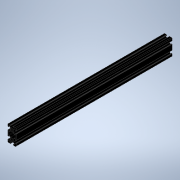
# Autodesk Inventor part: 2020 Aluminium Extrusion European Standard
Saved by Autodesk Inventor 2020 (Build 240168000, 168)
## iProperties
Created: 2019-10-16
Part Number: 2020 Aluminium Extrusion European Standard
Material: Generic
Document SubType Name: Modeling
Designer: Johnson Ebenezer R
Density: 1 g/cm^3
Appearance: Anodized - Black
Author: Johnson Ebenezer R
## iProperties of the stored document _3DPrint.ipt
Created: 2019-10-16
Part Number: _3DPrint
Material: Generic
Document SubType Name: Modeling
Designer: Johnson Ebenezer R
Density: 1 g/cm^3
Appearance: Default
Author: Johnson Ebenezer R
Autodesk Inventor part; units mm, degrees
ref_plane "YZ Plane" through (0, 0, 0) normal (1, 0, 0) x (0, 1, 0)
ref_plane "XZ Plane" through (0, 0, 0) normal (0, 1, 0) x (-1, 0, 0)
ref_plane "XY Plane" through (0, 0, 0) normal (0, 0, 1) x (1, 0, 0)
sketch "Sketch1" plane through (0, 0, 0) normal (0, 0, 1) x (1, 0, 0)
  line L0 (-10, -10) -> (10, -10) construction
  line L1 (10, -10) -> (10, 10) construction
  line L2 (10, 10) -> (-10, 10) construction
  line L3 (-10, 10) -> (-10, -10) construction
  line L4 (-10, -10) -> (10, 10) construction
  line L5 (10, -10) -> (-10, 10) construction
  line L6 (-10, 0) -> (10, 0) construction
  line L7 (-3.6, -10) -> (-10, -10)
  line L8 (-10, -10) -> (-10, -3.6)
  line L9 (3.6, -10) -> (10, -10)
  line L10 (10, -10) -> (10, -3.6)
  line L11 (-3.6, -10) -> (-3.6, -9.1)
  line L12 (3.6, -10) -> (3.6, -9.1)
  line L13 (-3.6, -9.1) -> (-3.1, -9.1)
  line L14 (-3.1, -9.1) -> (-3.1, -8.2)
  line L15 (3.6, -9.1) -> (3.1, -9.1)
  line L16 (3.1, -9.1) -> (3.1, -8.2)
  line L17 (-3.1, -8.2) -> (-5.45, -8.2)
  line L18 (-5.45, -8.2) -> (-5.45, -6.2985)
  line L19 (3.1, -8.2) -> (5.45, -8.2)
  line L20 (5.45, -8.2) -> (5.45, -6.2985)
  line L21 (-5.45, -6.2985) -> (-3.0515, -3.9)
  line L22 (-10, -3.6) -> (-9.1, -3.6)
  line L23 (-9.1, -3.6) -> (-9.1, -3.1)
  line L24 (-9.1, -3.1) -> (-8.2, -3.1)
  line L25 (-8.2, -3.1) -> (-8.2, -5.45)
  line L26 (-8.2, -5.45) -> (-6.2985, -5.45)
  line L27 (-6.2985, -5.45) -> (-3.9, -3.0515)
  circle A0 centre (0, 0) radius 2.5
  line L28 (5.45, -6.2985) -> (3.0515, -3.9)
  line L29 (3.0515, -3.9) -> (-3.0515, -3.9)
  line L30 (10, -3.6) -> (9.1, -3.6)
  line L31 (9.1, -3.6) -> (9.1, -3.1)
  line L32 (9.1, -3.1) -> (8.2, -3.1)
  line L33 (8.2, -3.1) -> (8.2, -5.45)
  line L34 (8.2, -5.45) -> (6.2985, -5.45)
  line L35 (6.2985, -5.45) -> (3.9485, -3.1)
  line L36 (-10, 10) -> (10, 10) construction
  line L37 (3.0515, 3.9) -> (-3.0515, 3.9)
  line L38 (-6.2985, 5.45) -> (-3.9, 3.0515)
  line L39 (-10, 10) -> (-10, 3.6)
  line L40 (-8.2, 3.1) -> (-8.2, 5.45)
  line L41 (-9.1, 3.1) -> (-8.2, 3.1)
  line L42 (-9.1, 3.6) -> (-9.1, 3.1)
  line L43 (-10, 3.6) -> (-9.1, 3.6)
  line L44 (-8.2, 5.45) -> (-6.2985, 5.45)
  line L45 (10, 10) -> (10, 3.6)
  line L46 (6.2985, 5.45) -> (3.9485, 3.1)
  line L47 (8.2, 5.45) -> (6.2985, 5.45)
  line L48 (8.2, 3.1) -> (8.2, 5.45)
  line L49 (9.1, 3.1) -> (8.2, 3.1)
  line L50 (9.1, 3.6) -> (9.1, 3.1)
  line L51 (10, 3.6) -> (9.1, 3.6)
  line L52 (-3.9, -3.0515) -> (-3.9, 3.0515)
  line L53 (3.9485, -3.1) -> (3.9485, 3.1)
  line L54 (-3.0515, 3.9) -> (-5.8015, 6.65)
  line L55 (3.0515, 3.9) -> (5.8015, 6.65)
  line L56 (-5.8015, 6.65) -> (-8.2, 6.65)
  line L57 (5.8015, 6.65) -> (8.2, 6.65)
  line L58 (-8.2, 6.65) -> (-8.2, 10)
  line L59 (8.2, 6.65) -> (8.2, 10)
  line L60 (-10, 30) -> (10, 30) construction
  line L61 (10, 30) -> (10, 10) construction
  line L62 (-10, 10) -> (-10, 30) construction
  line L63 (-10, 20) -> (10, 20) construction
  circle A1 centre (0, 20) radius 2.5
  line L64 (3.0515, 23.9) -> (-3.0515, 23.9)
  line L65 (-3.6, 30) -> (-3.6, 29.1)
  line L66 (-3.6, 29.1) -> (-3.1, 29.1)
  line L67 (-3.1, 29.1) -> (-3.1, 28.2)
  line L68 (-5.45, 26.2985) -> (-3.0515, 23.9)
  line L69 (-3.1, 28.2) -> (-5.45, 28.2)
  line L70 (-5.45, 28.2) -> (-5.45, 26.2985)
  line L71 (-6.2985, 25.45) -> (-3.9, 23.0515)
  line L72 (-3.6, 30) -> (-10, 30)
  line L73 (-10, 30) -> (-10, 23.6)
  line L74 (-8.2, 23.1) -> (-8.2, 25.45)
  line L75 (-9.1, 23.1) -> (-8.2, 23.1)
  line L76 (-9.1, 23.6) -> (-9.1, 23.1)
  line L77 (-10, 23.6) -> (-9.1, 23.6)
  line L78 (-8.2, 25.45) -> (-6.2985, 25.45)
  line L79 (3.6, 30) -> (10, 30)
  line L80 (10, 30) -> (10, 23.6)
  line L81 (3.6, 30) -> (3.6, 29.1)
  line L82 (3.6, 29.1) -> (3.1, 29.1)
  line L83 (3.1, 29.1) -> (3.1, 28.2)
  line L84 (3.1, 28.2) -> (5.45, 28.2)
  line L85 (5.45, 26.2985) -> (3.0515, 23.9)
  line L86 (5.45, 28.2) -> (5.45, 26.2985)
  line L87 (6.2985, 25.45) -> (3.9485, 23.1)
  line L88 (8.2, 25.45) -> (6.2985, 25.45)
  line L89 (8.2, 23.1) -> (8.2, 25.45)
  line L90 (9.1, 23.1) -> (8.2, 23.1)
  line L91 (9.1, 23.6) -> (9.1, 23.1)
  line L92 (10, 23.6) -> (9.1, 23.6)
  line L93 (3.0515, 16.1) -> (-3.0515, 16.1)
  line L94 (-6.2985, 14.55) -> (-3.9, 16.9485)
  line L95 (-8.2, 16.9) -> (-8.2, 14.55)
  line L96 (-8.2, 14.55) -> (-6.2985, 14.55)
  line L97 (-10, 10) -> (-10, 16.4)
  line L98 (-9.1, 16.9) -> (-8.2, 16.9)
  line L99 (-9.1, 16.4) -> (-9.1, 16.9)
  line L100 (-10, 16.4) -> (-9.1, 16.4)
  line L101 (6.2985, 14.55) -> (3.9485, 16.9)
  line L102 (8.2, 14.55) -> (6.2985, 14.55)
  line L103 (8.2, 16.9) -> (8.2, 14.55)
  line L104 (9.1, 16.9) -> (8.2, 16.9)
  line L105 (9.1, 16.4) -> (9.1, 16.9)
  line L106 (10, 10) -> (10, 16.4)
  line L107 (10, 16.4) -> (9.1, 16.4)
  line L108 (-3.9, 23.0515) -> (-3.9, 16.9485)
  line L109 (3.9485, 23.1) -> (3.9485, 16.9)
  line L110 (-3.0515, 16.1) -> (-5.8015, 13.35)
  line L111 (3.0515, 16.1) -> (5.8015, 13.35)
  line L112 (-5.8015, 13.35) -> (-8.2, 13.35)
  line L113 (5.8015, 13.35) -> (8.2, 13.35)
  line L114 (-8.2, 13.35) -> (-8.2, 10)
  line L115 (8.2, 13.35) -> (8.2, 10)
  point P0 (0, 0)
  point P1 (0, 0)
  point P2 (0, 20)
  point P3 (0, 20)
  dimension "len" = 20
  dimension "d1" = 20
  dimension "d2" = 7.2
  dimension "d3" = 0.9
  dimension "d4" = 6.2
  dimension "d5" = 1.8
  dimension "d6" = 10.9
  dimension "d8" = 5
  dimension "d9" = 6.1
  dimension "d13" = 1.2
  dimension "d19" = 1.2
  constraints: 232 end point, 72 symmetric about line, 21 equal length, 16 point on line, 14 perpendicular, 11 horizontal, 9 parallel, 5 midpoint, 4 coincident, 3 vertical, 2 centre point, 2 collinear, 1 other
  measures "len" distance of L1.end L2.end
  measures "d1" distance of L0.end L1.end
  measures "d2" distance of L9.start L11.start
  measures "d3" distance of L11.start L11.end
  measures "d4" distance of L15.end L13.end
  measures "d5" distance from line of L14.end L0
  measures "d6" distance between parallel lines of L20 L18
  measures "d8" diameter of A0
  measures "d9" distance between parallel lines of L29 L0
  measures "d13" distance between parallel lines of L27 L21
  measures "d19" distance between parallel lines of L56 L44
extrude "380mm" add sketch "Sketch1" along normal blind 380
fillet "Fillet 0.2mm" radius 0.2 12 edges at (-3.6, -9.1, 190) (3.6, -9.1, 190) (9.1, -3.6, 190) (-9.1, -3.6, 190) (-9.1, 3.6, 190) (9.1, 3.6, 190) (9.1, 16.4, 190) (9.1, 23.6, 190) (-9.1, 23.6, 190) (-9.1, 16.4, 190) (-3.6, 29.1, 190) (3.6, 29.1, 190)
fillet "Fillet 1.5mm" radius 1.5 4 edges at (-10, -10, 190) (10, -10, 190) (10, 30, 190) (-10, 30, 190)
equation "\"d1\" = len"
body "Solid1"
